Autodesk Fusion 360 part; units mm, degrees
(part 5 of 7)
sketch "Sketch2" plane through (0, 0, 2.4) normal (0, 0, 1) x (-1, 0, 0)
  circle A0 centre (0, 0) radius 8
  circle A1 centre (-15, 0) radius 5
  circle A2 centre (-4.6353, -14.2658) radius 5
  circle A3 centre (12.1353, -8.8168) radius 5
  circle A4 centre (12.1353, 8.8168) radius 5
  circle A5 centre (-4.6353, 14.2658) radius 5
  spline S0 degree 3 poles (-29.7434, 3.9157) (-29.7721, 3.6879) (-29.7146, 3.4878) (-29.6557, 3.3817) (-29.6311, 3.3373) (-29.6049, 3.3046) (-29.584, 3.2827) (-29.5723, 3.2703) (-29.5626, 3.2612) (-29.5043, 3.2074) (-29.4679, 3.1738) (-29.4161, 3.1342) (-29.3067, 3.0042) (-29.2288, 2.9117) (-29.097, 2.7401) (-29.0108, 2.4766) (-28.943, 2.2694) (-28.9321, 2.0574) (-28.9353, 1.9521) (-28.9382, 1.8554) (-28.9402, 1.7765) (-28.9853, 1.605) (-29.0418, 1.39) (-29.1868, 1.1346) (-29.3008, 0.9996) (-29.5122, 0.7494) (-29.5978, 0.7228) (-29.6536, 0.6831) (-29.7775, 0.595) (-29.758, 0.61) (-29.7843, 0.5851) (-29.8704, 0.5036) (-29.9984, 0.2947) (-30, -0.0001) knots 0.001251 0.001251 0.001251 0.001251 0.25 0.25 0.25 0.35404 0.35404 0.35404 0.412746 0.412746 0.412746 0.449449 0.449449 0.449449 0.475576 0.475576 0.475576 0.496118 0.496118 0.496118 0.514995 0.514995 0.514995 0.538647 0.538647 0.538647 0.582499 0.582499 0.582499 0.679826 0.679826 0.679826 0.99875 0.99875 0.99875 0.99875
  spline S1 degree 3 poles (-30, -0.0001) (-29.9988, -0.2297) (-29.9157, -0.4205) (-29.8434, -0.5181) (-29.8132, -0.5589) (-29.7829, -0.5878) (-29.7594, -0.6069) (-29.7462, -0.6177) (-29.7353, -0.6254) (-29.6705, -0.6711) (-29.63, -0.6997) (-29.5735, -0.7321) (-29.4481, -0.8468) (-29.3588, -0.9283) (-29.2058, -1.0812) (-29.0859, -1.3313) (-28.9916, -1.5279) (-28.9531, -1.7366) (-28.9425, -1.8414) (-28.9328, -1.9377) (-28.9245, -2.0161) (-28.9468, -2.1921) (-28.9748, -2.4126) (-29.0852, -2.6848) (-29.1806, -2.8335) (-29.3575, -3.1091) (-29.4389, -3.1467) (-29.4891, -3.1933) (-29.6004, -3.2968) (-29.583, -3.2795) (-29.6058, -3.3076) (-29.6806, -3.3996) (-29.7802, -3.6234) (-29.7433, -3.9159) knots 0.001251 0.001251 0.001251 0.001251 0.25 0.25 0.25 0.35404 0.35404 0.35404 0.412746 0.412746 0.412746 0.449449 0.449449 0.449449 0.475576 0.475576 0.475576 0.496118 0.496118 0.496118 0.514995 0.514995 0.514995 0.538647 0.538647 0.538647 0.582499 0.582499 0.582499 0.679826 0.679826 0.679826 0.99875 0.99875 0.99875 0.99875
  spline S2 degree 3 poles (-29.7433, -3.9159) (-29.7122, -4.1433) (-29.6048, -4.3217) (-29.5205, -4.409) (-29.4852, -4.4455) (-29.4514, -4.4703) (-29.4256, -4.4861) (-29.4111, -4.495) (-29.3993, -4.5013) (-29.3291, -4.5382) (-29.2852, -4.5612) (-29.2249, -4.586) (-29.0856, -4.6833) (-28.9864, -4.7525) (-28.8148, -4.8841) (-28.6632, -5.1164) (-28.5441, -5.299) (-28.4788, -5.5009) (-28.4546, -5.6034) (-28.4323, -5.6976) (-28.4139, -5.7743) (-28.413, -5.9517) (-28.412, -6.1739) (-28.4859, -6.4582) (-28.5611, -6.6181) (-28.7005, -6.9144) (-28.7764, -6.9623) (-28.82, -7.0151) (-28.9168, -7.1322) (-28.9019, -7.1128) (-28.9208, -7.1436) (-28.9829, -7.2446) (-29.0525, -7.4795) (-28.9777, -7.7647) knots 0.001251 0.001251 0.001251 0.001251 0.25 0.25 0.25 0.35404 0.35404 0.35404 0.412746 0.412746 0.412746 0.449449 0.449449 0.449449 0.475576 0.475576 0.475576 0.496118 0.496118 0.496118 0.514995 0.514995 0.514995 0.538647 0.538647 0.538647 0.582499 0.582499 0.582499 0.679826 0.679826 0.679826 0.99875 0.99875 0.99875 0.99875
  spline S3 degree 3 poles (-28.9777, -7.7647) (-28.9172, -7.9861) (-28.7875, -8.1489) (-28.6924, -8.2245) (-28.6527, -8.2561) (-28.616, -8.2762) (-28.5883, -8.2885) (-28.5727, -8.2955) (-28.5603, -8.3002) (-28.4858, -8.3276) (-28.4393, -8.3447) (-28.3763, -8.3614) (-28.2255, -8.4396) (-28.1181, -8.4953) (-27.9308, -8.6034) (-27.7502, -8.8139) (-27.6083, -8.9794) (-27.5171, -9.1711) (-27.4797, -9.2695) (-27.4454, -9.36) (-27.4171, -9.4336) (-27.3931, -9.6094) (-27.363, -9.8296) (-27.3993, -10.1211) (-27.4529, -10.2894) (-27.5525, -10.6015) (-27.6214, -10.6588) (-27.6578, -10.7168) (-27.7385, -10.8456) (-27.7262, -10.8244) (-27.741, -10.8574) (-27.7894, -10.9657) (-27.8277, -11.2076) (-27.7163, -11.4806) knots 0.001251 0.001251 0.001251 0.001251 0.25 0.25 0.25 0.35404 0.35404 0.35404 0.412746 0.412746 0.412746 0.449449 0.449449 0.449449 0.475576 0.475576 0.475576 0.496118 0.496118 0.496118 0.514995 0.514995 0.514995 0.538647 0.538647 0.538647 0.582499 0.582499 0.582499 0.679826 0.679826 0.679826 0.99875 0.99875 0.99875 0.99875
  spline S4 degree 3 poles (-27.7163, -11.4806) (-27.6274, -11.6922) (-27.4775, -11.8368) (-27.3735, -11.8992) (-27.3299, -11.9254) (-27.2909, -11.9405) (-27.2619, -11.9492) (-27.2455, -11.954) (-27.2325, -11.9571) (-27.1552, -11.9745) (-27.1068, -11.9853) (-27.0422, -11.9937) (-26.8824, -12.0516) (-26.7687, -12.0928) (-26.5688, -12.1755) (-26.3624, -12.3606) (-26.2, -12.5062) (-26.0846, -12.6843) (-26.0347, -12.7771) (-25.9889, -12.8623) (-25.9512, -12.9316) (-25.9045, -13.1027) (-25.8459, -13.3171) (-25.8438, -13.6108) (-25.875, -13.7847) (-25.933, -14.1071) (-25.9939, -14.173) (-26.0223, -14.2352) (-26.0856, -14.3734) (-26.0762, -14.3508) (-26.0865, -14.3854) (-26.1203, -14.4991) (-26.1267, -14.744) (-25.9807, -15.0001) knots 0.001251 0.001251 0.001251 0.001251 0.25 0.25 0.25 0.35404 0.35404 0.35404 0.412746 0.412746 0.412746 0.449449 0.449449 0.449449 0.475576 0.475576 0.475576 0.496118 0.496118 0.496118 0.514995 0.514995 0.514995 0.538647 0.538647 0.538647 0.582499 0.582499 0.582499 0.679826 0.679826 0.679826 0.99875 0.99875 0.99875 0.99875
  spline S5 degree 3 poles (-25.9807, -15.0001) (-25.8649, -15.1983) (-25.6975, -15.322) (-25.5861, -15.3704) (-25.5395, -15.3906) (-25.4989, -15.4006) (-25.469, -15.4053) (-25.4521, -15.408) (-25.4388, -15.4093) (-25.3599, -15.4165) (-25.3105, -15.421) (-25.2453, -15.4208) (-25.0794, -15.4573) (-24.9613, -15.4834) (-24.7523, -15.5393) (-24.5234, -15.6959) (-24.3435, -15.819) (-24.2058, -15.9805) (-24.1443, -16.066) (-24.0877, -16.1444) (-24.0413, -16.2082) (-23.9726, -16.3718) (-23.8866, -16.5767) (-23.8461, -16.8677) (-23.8544, -17.0441) (-23.8698, -17.3713) (-23.9215, -17.4446) (-23.9416, -17.51) (-23.9863, -17.6553) (-23.9799, -17.6316) (-23.9856, -17.6673) (-24.0044, -17.7844) (-23.9787, -18.028) (-23.8005, -18.2629) knots 0.001251 0.001251 0.001251 0.001251 0.25 0.25 0.25 0.35404 0.35404 0.35404 0.412746 0.412746 0.412746 0.449449 0.449449 0.449449 0.475576 0.475576 0.475576 0.496118 0.496118 0.496118 0.514995 0.514995 0.514995 0.538647 0.538647 0.538647 0.582499 0.582499 0.582499 0.679826 0.679826 0.679826 0.99875 0.99875 0.99875 0.99875
  spline S6 degree 3 poles (-23.8005, -18.2629) (-23.6598, -18.4443) (-23.4777, -18.5451) (-23.361, -18.5786) (-23.3122, -18.5925) (-23.2705, -18.5971) (-23.2403, -18.5979) (-23.2232, -18.5984) (-23.2099, -18.5979) (-23.1307, -18.5947) (-23.0811, -18.5927) (-23.0165, -18.5841) (-22.8472, -18.5986) (-22.7267, -18.609) (-22.5123, -18.6372) (-22.2649, -18.7625) (-22.0704, -18.8611) (-21.9129, -19.0033) (-21.8407, -19.08) (-21.7743, -19.1504) (-21.72, -19.2076) (-21.6306, -19.3608) (-21.5185, -19.5527) (-21.4404, -19.8359) (-21.4256, -20.012) (-21.3981, -20.3383) (-21.4399, -20.4177) (-21.4513, -20.4852) (-21.4766, -20.6351) (-21.4734, -20.6108) (-21.4744, -20.647) (-21.4777, -20.7655) (-21.4205, -21.0037) (-21.2131, -21.2133) knots 0.001251 0.001251 0.001251 0.001251 0.25 0.25 0.25 0.35404 0.35404 0.35404 0.412746 0.412746 0.412746 0.449449 0.449449 0.449449 0.475576 0.475576 0.475576 0.496118 0.496118 0.496118 0.514995 0.514995 0.514995 0.538647 0.538647 0.538647 0.582499 0.582499 0.582499 0.679826 0.679826 0.679826 0.99875 0.99875 0.99875 0.99875
  spline S7 degree 3 poles (-21.2131, -21.2133) (-21.05, -21.3747) (-20.8562, -21.4509) (-20.7361, -21.4688) (-20.6859, -21.4763) (-20.6441, -21.4754) (-20.6139, -21.4722) (-20.5969, -21.4705) (-20.5838, -21.4683) (-20.5057, -21.4548) (-20.4568, -21.4463) (-20.3939, -21.4293) (-20.2242, -21.4217) (-20.1033, -21.4162) (-19.887, -21.4162) (-19.6254, -21.5082) (-19.4198, -21.5805) (-19.245, -21.701) (-19.1634, -21.7675) (-19.0884, -21.8287) (-19.0271, -21.8783) (-18.9184, -22.0185) (-18.7823, -22.1942) (-18.6679, -22.4648) (-18.6302, -22.6374) (-18.5604, -22.9574) (-18.5914, -23.0415) (-18.5939, -23.1099) (-18.5994, -23.2618) (-18.5994, -23.2373) (-18.5957, -23.2733) (-18.5835, -23.3912) (-18.4957, -23.6199) (-18.2627, -23.8007) knots 0.001251 0.001251 0.001251 0.001251 0.25 0.25 0.25 0.35404 0.35404 0.35404 0.412746 0.412746 0.412746 0.449449 0.449449 0.449449 0.475576 0.475576 0.475576 0.496118 0.496118 0.496118 0.514995 0.514995 0.514995 0.538647 0.538647 0.538647 0.582499 0.582499 0.582499 0.679826 0.679826 0.679826 0.99875 0.99875 0.99875 0.99875
  spline S8 degree 3 poles (-18.2627, -23.8007) (-18.0799, -23.9394) (-17.8779, -23.9897) (-17.7565, -23.9918) (-17.7057, -23.9926) (-17.6643, -23.9862) (-17.6349, -23.9792) (-17.6183, -23.9752) (-17.6055, -23.9714) (-17.5298, -23.9478) (-17.4825, -23.933) (-17.4224, -23.908) (-17.2551, -23.8782) (-17.136, -23.857) (-16.9215, -23.8287) (-16.6502, -23.8858) (-16.4368, -23.9307) (-16.2478, -24.0273) (-16.1582, -24.0826) (-16.0759, -24.1335) (-16.0086, -24.1747) (-15.8826, -24.2995) (-15.7247, -24.4559) (-15.576, -24.7092) (-15.5161, -24.8754) (-15.4051, -25.1836) (-15.4249, -25.2711) (-15.4184, -25.3392) (-15.404, -25.4905) (-15.4072, -25.4662) (-15.3988, -25.5014) (-15.3713, -25.6167) (-15.2544, -25.832) (-14.9999, -25.9808) knots 0.001251 0.001251 0.001251 0.001251 0.25 0.25 0.25 0.35404 0.35404 0.35404 0.412746 0.412746 0.412746 0.449449 0.449449 0.449449 0.475576 0.475576 0.475576 0.496118 0.496118 0.496118 0.514995 0.514995 0.514995 0.538647 0.538647 0.538647 0.582499 0.582499 0.582499 0.679826 0.679826 0.679826 0.99875 0.99875 0.99875 0.99875
  spline S9 degree 3 poles (-14.9999, -25.9808) (-14.8005, -26.0945) (-14.5936, -26.118) (-14.473, -26.1042) (-14.4226, -26.0984) (-14.3824, -26.0867) (-14.3541, -26.0759) (-14.3382, -26.0698) (-14.326, -26.0643) (-14.2541, -26.031) (-14.2091, -26.0102) (-14.1527, -25.9775) (-13.9907, -25.9262) (-13.8754, -25.8896) (-13.6665, -25.8336) (-13.39, -25.8547) (-13.1726, -25.8714) (-12.9726, -25.9425) (-12.8766, -25.9857) (-12.7883, -26.0253) (-12.7162, -26.0574) (-12.575, -26.1647) (-12.398, -26.2992) (-12.2175, -26.5309) (-12.1364, -26.6879) (-11.9862, -26.9789) (-11.9944, -27.0682) (-11.9791, -27.135) (-11.9451, -27.2831) (-11.9514, -27.2594) (-11.9385, -27.2932) (-11.8962, -27.4039) (-11.7522, -27.6021) (-11.4804, -27.7164) knots 0.001251 0.001251 0.001251 0.001251 0.25 0.25 0.25 0.35404 0.35404 0.35404 0.412746 0.412746 0.412746 0.449449 0.449449 0.449449 0.475576 0.475576 0.475576 0.496118 0.496118 0.496118 0.514995 0.514995 0.514995 0.538647 0.538647 0.538647 0.582499 0.582499 0.582499 0.679826 0.679826 0.679826 0.99875 0.99875 0.99875 0.99875
  spline S10 degree 3 poles (-11.4804, -27.7164) (-11.2679, -27.8031) (-11.0597, -27.7994) (-10.9419, -27.77) (-10.8927, -27.7577) (-10.8543, -27.7408) (-10.8277, -27.7264) (-10.8127, -27.7182) (-10.8014, -27.7112) (-10.7344, -27.6688) (-10.6925, -27.6423) (-10.6409, -27.6025) (-10.487, -27.5305) (-10.3774, -27.4792) (-10.1776, -27.3964) (-9.9007, -27.3813) (-9.683, -27.3694) (-9.4754, -27.4138) (-9.3746, -27.4441) (-9.2819, -27.4719) (-9.2063, -27.4943) (-9.0522, -27.5822) (-8.8592, -27.6924) (-8.65, -27.8986) (-8.5492, -28.0437) (-8.3622, -28.3126) (-8.3586, -28.4022) (-8.3347, -28.4664) (-8.2817, -28.6088) (-8.2911, -28.5861) (-8.2739, -28.618) (-8.2175, -28.7223) (-8.0488, -28.8999) (-7.7644, -28.9778) knots 0.001251 0.001251 0.001251 0.001251 0.25 0.25 0.25 0.35404 0.35404 0.35404 0.412746 0.412746 0.412746 0.449449 0.449449 0.449449 0.475576 0.475576 0.475576 0.496118 0.496118 0.496118 0.514995 0.514995 0.514995 0.538647 0.538647 0.538647 0.582499 0.582499 0.582499 0.679826 0.679826 0.679826 0.99875 0.99875 0.99875 0.99875
  spline S11 degree 3 poles (-7.7644, -28.9778) (-7.5424, -29.036) (-7.3365, -29.0052) (-7.2236, -28.9606) (-7.1764, -28.942) (-7.1406, -28.9203) (-7.1161, -28.9025) (-7.1022, -28.8924) (-7.0919, -28.884) (-7.031, -28.8332) (-6.993, -28.8015) (-6.947, -28.7553) (-6.8038, -28.6638) (-6.7019, -28.5987) (-6.5146, -28.4905) (-6.242, -28.4393) (-6.0278, -28.3991) (-5.8162, -28.4161) (-5.7122, -28.4329) (-5.6167, -28.4484) (-5.5388, -28.4607) (-5.3746, -28.5278) (-5.1689, -28.6119) (-4.9345, -28.789) (-4.8156, -28.9196) (-4.5951, -29.1619) (-4.5799, -29.2503) (-4.5478, -29.3108) (-4.4767, -29.445) (-4.4889, -29.4238) (-4.4677, -29.4531) (-4.3982, -29.5491) (-4.2078, -29.7033) (-3.9157, -29.7434) knots 0.001251 0.001251 0.001251 0.001251 0.25 0.25 0.25 0.35404 0.35404 0.35404 0.412746 0.412746 0.412746 0.449449 0.449449 0.449449 0.475576 0.475576 0.475576 0.496118 0.496118 0.496118 0.514995 0.514995 0.514995 0.538647 0.538647 0.538647 0.582499 0.582499 0.582499 0.679826 0.679826 0.679826 0.99875 0.99875 0.99875 0.99875
  spline S12 degree 3 poles (-3.9157, -29.7434) (-3.6879, -29.7721) (-3.4878, -29.7146) (-3.3817, -29.6557) (-3.3373, -29.6311) (-3.3046, -29.6049) (-3.2827, -29.584) (-3.2703, -29.5723) (-3.2612, -29.5626) (-3.2074, -29.5043) (-3.1738, -29.4679) (-3.1342, -29.4161) (-3.0042, -29.3067) (-2.9117, -29.2288) (-2.7401, -29.097) (-2.4766, -29.0108) (-2.2694, -28.943) (-2.0574, -28.9321) (-1.9521, -28.9353) (-1.8554, -28.9382) (-1.7765, -28.9402) (-1.605, -28.9853) (-1.39, -29.0418) (-1.1346, -29.1868) (-0.9996, -29.3008) (-0.7494, -29.5122) (-0.7228, -29.5978) (-0.6831, -29.6536) (-0.595, -29.7775) (-0.61, -29.758) (-0.5851, -29.7843) (-0.5036, -29.8704) (-0.2947, -29.9984) (0.0001, -30) knots 0.001251 0.001251 0.001251 0.001251 0.25 0.25 0.25 0.35404 0.35404 0.35404 0.412746 0.412746 0.412746 0.449449 0.449449 0.449449 0.475576 0.475576 0.475576 0.496118 0.496118 0.496118 0.514995 0.514995 0.514995 0.538647 0.538647 0.538647 0.582499 0.582499 0.582499 0.679826 0.679826 0.679826 0.99875 0.99875 0.99875 0.99875
  spline S13 degree 3 poles (0.0001, -30) (0.2297, -29.9988) (0.4205, -29.9157) (0.5181, -29.8434) (0.5589, -29.8132) (0.5878, -29.7829) (0.6069, -29.7594) (0.6177, -29.7462) (0.6254, -29.7353) (0.6711, -29.6705) (0.6997, -29.63) (0.7321, -29.5735) (0.8468, -29.4481) (0.9283, -29.3588) (1.0812, -29.2058) (1.3313, -29.0859) (1.5279, -28.9916) (1.7366, -28.9531) (1.8414, -28.9425) (1.9377, -28.9328) (2.0161, -28.9245) (2.1921, -28.9468) (2.4126, -28.9748) (2.6848, -29.0852) (2.8335, -29.1806) (3.1091, -29.3575) (3.1467, -29.4389) (3.1933, -29.4891) (3.2968, -29.6004) (3.2795, -29.583) (3.3076, -29.6058) (3.3996, -29.6806) (3.6234, -29.7802) (3.9159, -29.7433) knots 0.001251 0.001251 0.001251 0.001251 0.25 0.25 0.25 0.35404 0.35404 0.35404 0.412746 0.412746 0.412746 0.449449 0.449449 0.449449 0.475576 0.475576 0.475576 0.496118 0.496118 0.496118 0.514995 0.514995 0.514995 0.538647 0.538647 0.538647 0.582499 0.582499 0.582499 0.679826 0.679826 0.679826 0.99875 0.99875 0.99875 0.99875
  spline S14 degree 3 poles (3.9159, -29.7433) (4.1433, -29.7122) (4.3217, -29.6048) (4.409, -29.5205) (4.4455, -29.4852) (4.4703, -29.4514) (4.4861, -29.4256) (4.495, -29.4111) (4.5013, -29.3993) (4.5382, -29.3291) (4.5612, -29.2852) (4.586, -29.2249) (4.6833, -29.0856) (4.7525, -28.9864) (4.8841, -28.8148) (5.1164, -28.6632) (5.299, -28.5441) (5.5009, -28.4788) (5.6034, -28.4546) (5.6976, -28.4323) (5.7743, -28.4139) (5.9517, -28.413) (6.1739, -28.412) (6.4582, -28.4859) (6.6181, -28.5611) (6.9144, -28.7005) (6.9623, -28.7764) (7.0151, -28.82) (7.1322, -28.9168) (7.1128, -28.9019) (7.1436, -28.9208) (7.2446, -28.9829) (7.4795, -29.0525) (7.7647, -28.9777) knots 0.001251 0.001251 0.001251 0.001251 0.25 0.25 0.25 0.35404 0.35404 0.35404 0.412746 0.412746 0.412746 0.449449 0.449449 0.449449 0.475576 0.475576 0.475576 0.496118 0.496118 0.496118 0.514995 0.514995 0.514995 0.538647 0.538647 0.538647 0.582499 0.582499 0.582499 0.679826 0.679826 0.679826 0.99875 0.99875 0.99875 0.99875
  spline S15 degree 3 poles (7.7647, -28.9777) (7.9861, -28.9172) (8.1489, -28.7875) (8.2245, -28.6924) (8.2561, -28.6527) (8.2762, -28.616) (8.2885, -28.5883) (8.2955, -28.5727) (8.3002, -28.5603) (8.3276, -28.4858) (8.3447, -28.4393) (8.3614, -28.3763) (8.4396, -28.2255) (8.4953, -28.1181) (8.6034, -27.9308) (8.8139, -27.7502) (8.9794, -27.6083) (9.1711, -27.5171) (9.2695, -27.4797) (9.36, -27.4454) (9.4336, -27.4171) (9.6094, -27.3931) (9.8296, -27.363) (10.1211, -27.3993) (10.2894, -27.4529) (10.6015, -27.5525) (10.6588, -27.6214) (10.7168, -27.6578) (10.8456, -27.7385) (10.8244, -27.7262) (10.8574, -27.741) (10.9657, -27.7894) (11.2076, -27.8277) (11.4806, -27.7163) knots 0.001251 0.001251 0.001251 0.001251 0.25 0.25 0.25 0.35404 0.35404 0.35404 0.412746 0.412746 0.412746 0.449449 0.449449 0.449449 0.475576 0.475576 0.475576 0.496118 0.496118 0.496118 0.514995 0.514995 0.514995 0.538647 0.538647 0.538647 0.582499 0.582499 0.582499 0.679826 0.679826 0.679826 0.99875 0.99875 0.99875 0.99875
  spline S16 degree 3 poles (11.4806, -27.7163) (11.6922, -27.6274) (11.8368, -27.4775) (11.8992, -27.3735) (11.9254, -27.3299) (11.9405, -27.2909) (11.9492, -27.2619) (11.954, -27.2455) (11.9571, -27.2325) (11.9745, -27.1552) (11.9853, -27.1068) (11.9937, -27.0422) (12.0516, -26.8824) (12.0928, -26.7687) (12.1755, -26.5688) (12.3606, -26.3624) (12.5062, -26.2) (12.6843, -26.0846) (12.7771, -26.0347) (12.8623, -25.9889) (12.9316, -25.9512) (13.1027, -25.9045) (13.3171, -25.8459) (13.6108, -25.8438) (13.7847, -25.875) (14.1071, -25.933) (14.173, -25.9939) (14.2352, -26.0223) (14.3734, -26.0856) (14.3508, -26.0762) (14.3854, -26.0865) (14.4991, -26.1203) (14.744, -26.1267) (15.0001, -25.9807) knots 0.001251 0.001251 0.001251 0.001251 0.25 0.25 0.25 0.35404 0.35404 0.35404 0.412746 0.412746 0.412746 0.449449 0.449449 0.449449 0.475576 0.475576 0.475576 0.496118 0.496118 0.496118 0.514995 0.514995 0.514995 0.538647 0.538647 0.538647 0.582499 0.582499 0.582499 0.679826 0.679826 0.679826 0.99875 0.99875 0.99875 0.99875
  spline S17 degree 3 poles (15.0001, -25.9807) (15.1983, -25.8649) (15.322, -25.6975) (15.3704, -25.5861) (15.3906, -25.5395) (15.4006, -25.4989) (15.4053, -25.469) (15.408, -25.4521) (15.4093, -25.4388) (15.4165, -25.3599) (15.421, -25.3105) (15.4208, -25.2453) (15.4573, -25.0794) (15.4834, -24.9613) (15.5393, -24.7523) (15.6959, -24.5234) (15.819, -24.3435) (15.9805, -24.2058) (16.066, -24.1443) (16.1444, -24.0877) (16.2082, -24.0413) (16.3718, -23.9726) (16.5767, -23.8866) (16.8677, -23.8461) (17.0441, -23.8544) (17.3713, -23.8698) (17.4446, -23.9215) (17.51, -23.9416) (17.6553, -23.9863) (17.6316, -23.9799) (17.6673, -23.9856) (17.7844, -24.0044) (18.028, -23.9787) (18.2629, -23.8005) knots 0.001251 0.001251 0.001251 0.001251 0.25 0.25 0.25 0.35404 0.35404 0.35404 0.412746 0.412746 0.412746 0.449449 0.449449 0.449449 0.475576 0.475576 0.475576 0.496118 0.496118 0.496118 0.514995 0.514995 0.514995 0.538647 0.538647 0.538647 0.582499 0.582499 0.582499 0.679826 0.679826 0.679826 0.99875 0.99875 0.99875 0.99875
  spline S18 degree 3 poles (18.2629, -23.8005) (18.4443, -23.6598) (18.5451, -23.4777) (18.5786, -23.361) (18.5925, -23.3122) (18.5971, -23.2705) (18.5979, -23.2403) (18.5984, -23.2232) (18.5979, -23.2099) (18.5947, -23.1307) (18.5927, -23.0811) (18.5841, -23.0165) (18.5986, -22.8472) (18.609, -22.7267) (18.6372, -22.5123) (18.7625, -22.2649) (18.8611, -22.0704) (19.0033, -21.9129) (19.08, -21.8407) (19.1504, -21.7743) (19.2076, -21.72) (19.3608, -21.6306) (19.5527, -21.5185) (19.8359, -21.4404) (20.012, -21.4256) (20.3383, -21.3981) (20.4177, -21.4399) (20.4852, -21.4513) (20.6351, -21.4766) (20.6108, -21.4734) (20.647, -21.4744) (20.7655, -21.4777) (21.0037, -21.4205) (21.2133, -21.2131) knots 0.001251 0.001251 0.001251 0.001251 0.25 0.25 0.25 0.35404 0.35404 0.35404 0.412746 0.412746 0.412746 0.449449 0.449449 0.449449 0.475576 0.475576 0.475576 0.496118 0.496118 0.496118 0.514995 0.514995 0.514995 0.538647 0.538647 0.538647 0.582499 0.582499 0.582499 0.679826 0.679826 0.679826 0.99875 0.99875 0.99875 0.99875
  spline S19 degree 3 poles (21.2133, -21.2131) (21.3747, -21.05) (21.4509, -20.8562) (21.4688, -20.7361) (21.4763, -20.6859) (21.4754, -20.6441) (21.4722, -20.6139) (21.4705, -20.5969) (21.4683, -20.5838) (21.4548, -20.5057) (21.4463, -20.4568) (21.4293, -20.3939) (21.4217, -20.2242) (21.4162, -20.1033) (21.4162, -19.887) (21.5082, -19.6254) (21.5805, -19.4198) (21.701, -19.245) (21.7675, -19.1634) (21.8287, -19.0884) (21.8783, -19.0271) (22.0185, -18.9184) (22.1942, -18.7823) (22.4648, -18.6679) (22.6374, -18.6302) (22.9574, -18.5604) (23.0415, -18.5914) (23.1099, -18.5939) (23.2618, -18.5994) (23.2373, -18.5994) (23.2733, -18.5957) (23.3912, -18.5835) (23.6199, -18.4957) (23.8007, -18.2627) knots 0.001251 0.001251 0.001251 0.001251 0.25 0.25 0.25 0.35404 0.35404 0.35404 0.412746 0.412746 0.412746 0.449449 0.449449 0.449449 0.475576 0.475576 0.475576 0.496118 0.496118 0.496118 0.514995 0.514995 0.514995 0.538647 0.538647 0.538647 0.582499 0.582499 0.582499 0.679826 0.679826 0.679826 0.99875 0.99875 0.99875 0.99875
  spline S20 degree 3 poles (23.8007, -18.2627) (23.9394, -18.0799) (23.9897, -17.8779) (23.9918, -17.7565) (23.9926, -17.7057) (23.9862, -17.6643) (23.9792, -17.6349) (23.9752, -17.6183) (23.9714, -17.6055) (23.9478, -17.5298) (23.933, -17.4825) (23.908, -17.4224) (23.8782, -17.2551) (23.857, -17.136) (23.8287, -16.9215) (23.8858, -16.6502) (23.9307, -16.4368) (24.0273, -16.2478) (24.0826, -16.1582) (24.1335, -16.0759) (24.1747, -16.0086) (24.2995, -15.8826) (24.4559, -15.7247) (24.7092, -15.576) (24.8754, -15.5161) (25.1836, -15.4051) (25.2711, -15.4249) (25.3392, -15.4184) (25.4905, -15.404) (25.4662, -15.4072) (25.5014, -15.3988) (25.6167, -15.3713) (25.832, -15.2544) (25.9808, -14.9999) knots 0.001251 0.001251 0.001251 0.001251 0.25 0.25 0.25 0.35404 0.35404 0.35404 0.412746 0.412746 0.412746 0.449449 0.449449 0.449449 0.475576 0.475576 0.475576 0.496118 0.496118 0.496118 0.514995 0.514995 0.514995 0.538647 0.538647 0.538647 0.582499 0.582499 0.582499 0.679826 0.679826 0.679826 0.99875 0.99875 0.99875 0.99875
  spline S21 degree 3 poles (25.9808, -14.9999) (26.0945, -14.8005) (26.118, -14.5936) (26.1042, -14.473) (26.0984, -14.4226) (26.0867, -14.3824) (26.0759, -14.3541) (26.0698, -14.3382) (26.0643, -14.326) (26.031, -14.2541) (26.0102, -14.2091) (25.9775, -14.1527) (25.9262, -13.9907) (25.8896, -13.8754) (25.8336, -13.6665) (25.8547, -13.39) (25.8714, -13.1726) (25.9425, -12.9726) (25.9857, -12.8766) (26.0253, -12.7883) (26.0574, -12.7162) (26.1647, -12.575) (26.2992, -12.398) (26.5309, -12.2175) (26.6879, -12.1364) (26.9789, -11.9862) (27.0682, -11.9944) (27.135, -11.9791) (27.2831, -11.9451) (27.2594, -11.9514) (27.2932, -11.9385) (27.4039, -11.8962) (27.6021, -11.7522) (27.7164, -11.4804) knots 0.001251 0.001251 0.001251 0.001251 0.25 0.25 0.25 0.35404 0.35404 0.35404 0.412746 0.412746 0.412746 0.449449 0.449449 0.449449 0.475576 0.475576 0.475576 0.496118 0.496118 0.496118 0.514995 0.514995 0.514995 0.538647 0.538647 0.538647 0.582499 0.582499 0.582499 0.679826 0.679826 0.679826 0.99875 0.99875 0.99875 0.99875
  spline S22 degree 3 poles (27.7164, -11.4804) (27.8031, -11.2679) (27.7994, -11.0597) (27.77, -10.9419) (27.7577, -10.8927) (27.7408, -10.8543) (27.7264, -10.8277) (27.7182, -10.8127) (27.7112, -10.8014) (27.6688, -10.7344) (27.6423, -10.6925) (27.6025, -10.6409) (27.5305, -10.487) (27.4792, -10.3774) (27.3964, -10.1776) (27.3813, -9.9007) (27.3694, -9.683) (27.4138, -9.4754) (27.4441, -9.3746) (27.4719, -9.2819) (27.4943, -9.2063) (27.5822, -9.0522) (27.6924, -8.8592) (27.8986, -8.65) (28.0437, -8.5492) (28.3126, -8.3622) (28.4022, -8.3586) (28.4664, -8.3347) (28.6088, -8.2817) (28.5861, -8.2911) (28.618, -8.2739) (28.7223, -8.2175) (28.8999, -8.0488) (28.9778, -7.7644) knots 0.001251 0.001251 0.001251 0.001251 0.25 0.25 0.25 0.35404 0.35404 0.35404 0.412746 0.412746 0.412746 0.449449 0.449449 0.449449 0.475576 0.475576 0.475576 0.496118 0.496118 0.496118 0.514995 0.514995 0.514995 0.538647 0.538647 0.538647 0.582499 0.582499 0.582499 0.679826 0.679826 0.679826 0.99875 0.99875 0.99875 0.99875
  spline S23 degree 3 poles (28.9778, -7.7644) (29.036, -7.5424) (29.0052, -7.3365) (28.9606, -7.2236) (28.942, -7.1764) (28.9203, -7.1406) (28.9025, -7.1161) (28.8924, -7.1022) (28.884, -7.0919) (28.8332, -7.031) (28.8015, -6.993) (28.7553, -6.947) (28.6638, -6.8038) (28.5987, -6.7019) (28.4905, -6.5146) (28.4393, -6.242) (28.3991, -6.0278) (28.4161, -5.8162) (28.4329, -5.7122) (28.4484, -5.6167) (28.4607, -5.5388) (28.5278, -5.3746) (28.6119, -5.1689) (28.789, -4.9345) (28.9196, -4.8156) (29.1619, -4.5951) (29.2503, -4.5799) (29.3108, -4.5478) (29.445, -4.4767) (29.4238, -4.4889) (29.4531, -4.4677) (29.5491, -4.3982) (29.7033, -4.2078) (29.7434, -3.9157) knots 0.001251 0.001251 0.001251 0.001251 0.25 0.25 0.25 0.35404 0.35404 0.35404 0.412746 0.412746 0.412746 0.449449 0.449449 0.449449 0.475576 0.475576 0.475576 0.496118 0.496118 0.496118 0.514995 0.514995 0.514995 0.538647 0.538647 0.538647 0.582499 0.582499 0.582499 0.679826 0.679826 0.679826 0.99875 0.99875 0.99875 0.99875
  spline S24 degree 3 poles (29.7434, -3.9157) (29.7721, -3.6879) (29.7146, -3.4878) (29.6557, -3.3817) (29.6311, -3.3373) (29.6049, -3.3046) (29.584, -3.2827) (29.5723, -3.2703) (29.5626, -3.2612) (29.5043, -3.2074) (29.4679, -3.1738) (29.4161, -3.1342) (29.3067, -3.0042) (29.2288, -2.9117) (29.097, -2.7401) (29.0108, -2.4766) (28.943, -2.2694) (28.9321, -2.0574) (28.9353, -1.9521) (28.9382, -1.8554) (28.9402, -1.7765) (28.9853, -1.605) (29.0418, -1.39) (29.1868, -1.1346) (29.3008, -0.9996) (29.5122, -0.7494) (29.5978, -0.7228) (29.6536, -0.6831) (29.7775, -0.595) (29.758, -0.61) (29.7843, -0.5851) (29.8704, -0.5036) (29.9984, -0.2947) (30, 0.0001) knots 0.001251 0.001251 0.001251 0.001251 0.25 0.25 0.25 0.35404 0.35404 0.35404 0.412746 0.412746 0.412746 0.449449 0.449449 0.449449 0.475576 0.475576 0.475576 0.496118 0.496118 0.496118 0.514995 0.514995 0.514995 0.538647 0.538647 0.538647 0.582499 0.582499 0.582499 0.679826 0.679826 0.679826 0.99875 0.99875 0.99875 0.99875
  spline S25 degree 3 poles (30, 0.0001) (29.9988, 0.2297) (29.9157, 0.4205) (29.8434, 0.5181) (29.8132, 0.5589) (29.7829, 0.5878) (29.7594, 0.6069) (29.7462, 0.6177) (29.7353, 0.6254) (29.6705, 0.6711) (29.63, 0.6997) (29.5735, 0.7321) (29.4481, 0.8468) (29.3588, 0.9283) (29.2058, 1.0812) (29.0859, 1.3313) (28.9916, 1.5279) (28.9531, 1.7366) (28.9425, 1.8414) (28.9328, 1.9377) (28.9245, 2.0161) (28.9468, 2.1921) (28.9748, 2.4126) (29.0852, 2.6848) (29.1806, 2.8335) (29.3575, 3.1091) (29.4389, 3.1467) (29.4891, 3.1933) (29.6004, 3.2968) (29.583, 3.2795) (29.6058, 3.3076) (29.6806, 3.3996) (29.7802, 3.6234) (29.7433, 3.9159) knots 0.001251 0.001251 0.001251 0.001251 0.25 0.25 0.25 0.35404 0.35404 0.35404 0.412746 0.412746 0.412746 0.449449 0.449449 0.449449 0.475576 0.475576 0.475576 0.496118 0.496118 0.496118 0.514995 0.514995 0.514995 0.538647 0.538647 0.538647 0.582499 0.582499 0.582499 0.679826 0.679826 0.679826 0.99875 0.99875 0.99875 0.99875
  spline S26 degree 3 poles (29.7433, 3.9159) (29.7122, 4.1433) (29.6048, 4.3217) (29.5205, 4.409) (29.4852, 4.4455) (29.4514, 4.4703) (29.4256, 4.4861) (29.4111, 4.495) (29.3993, 4.5013) (29.3291, 4.5382) (29.2852, 4.5612) (29.2249, 4.586) (29.0856, 4.6833) (28.9864, 4.7525) (28.8148, 4.8841) (28.6632, 5.1164) (28.5441, 5.299) (28.4788, 5.5009) (28.4546, 5.6034) (28.4323, 5.6976) (28.4139, 5.7743) (28.413, 5.9517) (28.412, 6.1739) (28.4859, 6.4582) (28.5611, 6.6181) (28.7005, 6.9144) (28.7764, 6.9623) (28.82, 7.0151) (28.9168, 7.1322) (28.9019, 7.1128) (28.9208, 7.1436) (28.9829, 7.2446) (29.0525, 7.4795) (28.9777, 7.7647) knots 0.001251 0.001251 0.001251 0.001251 0.25 0.25 0.25 0.35404 0.35404 0.35404 0.412746 0.412746 0.412746 0.449449 0.449449 0.449449 0.475576 0.475576 0.475576 0.496118 0.496118 0.496118 0.514995 0.514995 0.514995 0.538647 0.538647 0.538647 0.582499 0.582499 0.582499 0.679826 0.679826 0.679826 0.99875 0.99875 0.99875 0.99875
  spline S27 degree 3 poles (28.9777, 7.7647) (28.9172, 7.9861) (28.7875, 8.1489) (28.6924, 8.2245) (28.6527, 8.2561) (28.616, 8.2762) (28.5883, 8.2885) (28.5727, 8.2955) (28.5603, 8.3002) (28.4858, 8.3276) (28.4393, 8.3447) (28.3763, 8.3614) (28.2255, 8.4396) (28.1181, 8.4953) (27.9308, 8.6034) (27.7502, 8.8139) (27.6083, 8.9794) (27.5171, 9.1711) (27.4797, 9.2695) (27.4454, 9.36) (27.4171, 9.4336) (27.3931, 9.6094) (27.363, 9.8296) (27.3993, 10.1211) (27.4529, 10.2894) (27.5525, 10.6015) (27.6214, 10.6588) (27.6578, 10.7168) (27.7385, 10.8456) (27.7262, 10.8244) (27.741, 10.8574) (27.7894, 10.9657) (27.8277, 11.2076) (27.7163, 11.4806) knots 0.001251 0.001251 0.001251 0.001251 0.25 0.25 0.25 0.35404 0.35404 0.35404 0.412746 0.412746 0.412746 0.449449 0.449449 0.449449 0.475576 0.475576 0.475576 0.496118 0.496118 0.496118 0.514995 0.514995 0.514995 0.538647 0.538647 0.538647 0.582499 0.582499 0.582499 0.679826 0.679826 0.679826 0.99875 0.99875 0.99875 0.99875
  spline S28 degree 3 poles (27.7163, 11.4806) (27.6274, 11.6922) (27.4775, 11.8368) (27.3735, 11.8992) (27.3299, 11.9254) (27.2909, 11.9405) (27.2619, 11.9492) (27.2455, 11.954) (27.2325, 11.9571) (27.1552, 11.9745) (27.1068, 11.9853) (27.0422, 11.9937) (26.8824, 12.0516) (26.7687, 12.0928) (26.5688, 12.1755) (26.3624, 12.3606) (26.2, 12.5062) (26.0846, 12.6843) (26.0347, 12.7771) (25.9889, 12.8623) (25.9512, 12.9316) (25.9045, 13.1027) (25.8459, 13.3171) (25.8438, 13.6108) (25.875, 13.7847) (25.933, 14.1071) (25.9939, 14.173) (26.0223, 14.2352) (26.0856, 14.3734) (26.0762, 14.3508) (26.0865, 14.3854) (26.1203, 14.4991) (26.1267, 14.744) (25.9807, 15.0001) knots 0.001251 0.001251 0.001251 0.001251 0.25 0.25 0.25 0.35404 0.35404 0.35404 0.412746 0.412746 0.412746 0.449449 0.449449 0.449449 0.475576 0.475576 0.475576 0.496118 0.496118 0.496118 0.514995 0.514995 0.514995 0.538647 0.538647 0.538647 0.582499 0.582499 0.582499 0.679826 0.679826 0.679826 0.99875 0.99875 0.99875 0.99875
  spline S29 degree 3 poles (25.9807, 15.0001) (25.8649, 15.1983) (25.6975, 15.322) (25.5861, 15.3704) (25.5395, 15.3906) (25.4989, 15.4006) (25.469, 15.4053) (25.4521, 15.408) (25.4388, 15.4093) (25.3599, 15.4165) (25.3105, 15.421) (25.2453, 15.4208) (25.0794, 15.4573) (24.9613, 15.4834) (24.7523, 15.5393) (24.5234, 15.6959) (24.3435, 15.819) (24.2058, 15.9805) (24.1443, 16.066) (24.0877, 16.1444) (24.0413, 16.2082) (23.9726, 16.3718) (23.8866, 16.5767) (23.8461, 16.8677) (23.8544, 17.0441) (23.8698, 17.3713) (23.9215, 17.4446) (23.9416, 17.51) (23.9863, 17.6553) (23.9799, 17.6316) (23.9856, 17.6673) (24.0044, 17.7844) (23.9787, 18.028) (23.8005, 18.2629) knots 0.001251 0.001251 0.001251 0.001251 0.25 0.25 0.25 0.35404 0.35404 0.35404 0.412746 0.412746 0.412746 0.449449 0.449449 0.449449 0.475576 0.475576 0.475576 0.496118 0.496118 0.496118 0.514995 0.514995 0.514995 0.538647 0.538647 0.538647 0.582499 0.582499 0.582499 0.679826 0.679826 0.679826 0.99875 0.99875 0.99875 0.99875
  spline S30 degree 3 poles (23.8005, 18.2629) (23.6598, 18.4443) (23.4777, 18.5451) (23.361, 18.5786) (23.3122, 18.5925) (23.2705, 18.5971) (23.2403, 18.5979) (23.2232, 18.5984) (23.2099, 18.5979) (23.1307, 18.5947) (23.0811, 18.5927) (23.0165, 18.5841) (22.8472, 18.5986) (22.7267, 18.609) (22.5123, 18.6372) (22.2649, 18.7625) (22.0704, 18.8611) (21.9129, 19.0033) (21.8407, 19.08) (21.7743, 19.1504) (21.72, 19.2076) (21.6306, 19.3608) (21.5185, 19.5527) (21.4404, 19.8359) (21.4256, 20.012) (21.3981, 20.3383) (21.4399, 20.4177) (21.4513, 20.4852) (21.4766, 20.6351) (21.4734, 20.6108) (21.4744, 20.647) (21.4777, 20.7655) (21.4205, 21.0037) (21.2131, 21.2133) knots 0.001251 0.001251 0.001251 0.001251 0.25 0.25 0.25 0.35404 0.35404 0.35404 0.412746 0.412746 0.412746 0.449449 0.449449 0.449449 0.475576 0.475576 0.475576 0.496118 0.496118 0.496118 0.514995 0.514995 0.514995 0.538647 0.538647 0.538647 0.582499 0.582499 0.582499 0.679826 0.679826 0.679826 0.99875 0.99875 0.99875 0.99875
  spline S31 degree 3 poles (21.2131, 21.2133) (21.05, 21.3747) (20.8562, 21.4509) (20.7361, 21.4688) (20.6859, 21.4763) (20.6441, 21.4754) (20.6139, 21.4722) (20.5969, 21.4705) (20.5838, 21.4683) (20.5057, 21.4548) (20.4568, 21.4463) (20.3939, 21.4293) (20.2242, 21.4217) (20.1033, 21.4162) (19.887, 21.4162) (19.6254, 21.5082) (19.4198, 21.5805) (19.245, 21.701) (19.1634, 21.7675) (19.0884, 21.8287) (19.0271, 21.8783) (18.9184, 22.0185) (18.7823, 22.1942) (18.6679, 22.4648) (18.6302, 22.6374) (18.5604, 22.9574) (18.5914, 23.0415) (18.5939, 23.1099) (18.5994, 23.2618) (18.5994, 23.2373) (18.5957, 23.2733) (18.5835, 23.3912) (18.4957, 23.6199) (18.2627, 23.8007) knots 0.001251 0.001251 0.001251 0.001251 0.25 0.25 0.25 0.35404 0.35404 0.35404 0.412746 0.412746 0.412746 0.449449 0.449449 0.449449 0.475576 0.475576 0.475576 0.496118 0.496118 0.496118 0.514995 0.514995 0.514995 0.538647 0.538647 0.538647 0.582499 0.582499 0.582499 0.679826 0.679826 0.679826 0.99875 0.99875 0.99875 0.99875
  spline S32 degree 3 poles (18.2627, 23.8007) (18.0799, 23.9394) (17.8779, 23.9897) (17.7565, 23.9918) (17.7057, 23.9926) (17.6643, 23.9862) (17.6349, 23.9792) (17.6183, 23.9752) (17.6055, 23.9714) (17.5298, 23.9478) (17.4825, 23.933) (17.4224, 23.908) (17.2551, 23.8782) (17.136, 23.857) (16.9215, 23.8287) (16.6502, 23.8858) (16.4368, 23.9307) (16.2478, 24.0273) (16.1582, 24.0826) (16.0759, 24.1335) (16.0086, 24.1747) (15.8826, 24.2995) (15.7247, 24.4559) (15.576, 24.7092) (15.5161, 24.8754) (15.4051, 25.1836) (15.4249, 25.2711) (15.4184, 25.3392) (15.404, 25.4905) (15.4072, 25.4662) (15.3988, 25.5014) (15.3713, 25.6167) (15.2544, 25.832) (14.9999, 25.9808) knots 0.001251 0.001251 0.001251 0.001251 0.25 0.25 0.25 0.35404 0.35404 0.35404 0.412746 0.412746 0.412746 0.449449 0.449449 0.449449 0.475576 0.475576 0.475576 0.496118 0.496118 0.496118 0.514995 0.514995 0.514995 0.538647 0.538647 0.538647 0.582499 0.582499 0.582499 0.679826 0.679826 0.679826 0.99875 0.99875 0.99875 0.99875
  spline S33 degree 3 poles (14.9999, 25.9808) (14.8005, 26.0945) (14.5936, 26.118) (14.473, 26.1042) (14.4226, 26.0984) (14.3824, 26.0867) (14.3541, 26.0759) (14.3382, 26.0698) (14.326, 26.0643) (14.2541, 26.031) (14.2091, 26.0102) (14.1527, 25.9775) (13.9907, 25.9262) (13.8754, 25.8896) (13.6665, 25.8336) (13.39, 25.8547) (13.1726, 25.8714) (12.9726, 25.9425) (12.8766, 25.9857) (12.7883, 26.0253) (12.7162, 26.0574) (12.575, 26.1647) (12.398, 26.2992) (12.2175, 26.5309) (12.1364, 26.6879) (11.9862, 26.9789) (11.9944, 27.0682) (11.9791, 27.135) (11.9451, 27.2831) (11.9514, 27.2594) (11.9385, 27.2932) (11.8962, 27.4039) (11.7522, 27.6021) (11.4804, 27.7164) knots 0.001251 0.001251 0.001251 0.001251 0.25 0.25 0.25 0.35404 0.35404 0.35404 0.412746 0.412746 0.412746 0.449449 0.449449 0.449449 0.475576 0.475576 0.475576 0.496118 0.496118 0.496118 0.514995 0.514995 0.514995 0.538647 0.538647 0.538647 0.582499 0.582499 0.582499 0.679826 0.679826 0.679826 0.99875 0.99875 0.99875 0.99875
  spline S34 degree 3 poles (11.4804, 27.7164) (11.2679, 27.8031) (11.0597, 27.7994) (10.9419, 27.77) (10.8927, 27.7577) (10.8543, 27.7408) (10.8277, 27.7264) (10.8127, 27.7182) (10.8014, 27.7112) (10.7344, 27.6688) (10.6925, 27.6423) (10.6409, 27.6025) (10.487, 27.5305) (10.3774, 27.4792) (10.1776, 27.3964) (9.9007, 27.3813) (9.683, 27.3694) (9.4754, 27.4138) (9.3746, 27.4441) (9.2819, 27.4719) (9.2063, 27.4943) (9.0522, 27.5822) (8.8592, 27.6924) (8.65, 27.8986) (8.5492, 28.0437) (8.3622, 28.3126) (8.3586, 28.4022) (8.3347, 28.4664) (8.2817, 28.6088) (8.2911, 28.5861) (8.2739, 28.618) (8.2175, 28.7223) (8.0488, 28.8999) (7.7644, 28.9778) knots 0.001251 0.001251 0.001251 0.001251 0.25 0.25 0.25 0.35404 0.35404 0.35404 0.412746 0.412746 0.412746 0.449449 0.449449 0.449449 0.475576 0.475576 0.475576 0.496118 0.496118 0.496118 0.514995 0.514995 0.514995 0.538647 0.538647 0.538647 0.582499 0.582499 0.582499 0.679826 0.679826 0.679826 0.99875 0.99875 0.99875 0.99875
  spline S35 degree 3 poles (7.7644, 28.9778) (7.5424, 29.036) (7.3365, 29.0052) (7.2236, 28.9606) (7.1764, 28.942) (7.1406, 28.9203) (7.1161, 28.9025) (7.1022, 28.8924) (7.0919, 28.884) (7.031, 28.8332) (6.993, 28.8015) (6.947, 28.7553) (6.8038, 28.6638) (6.7019, 28.5987) (6.5146, 28.4905) (6.242, 28.4393) (6.0278, 28.3991) (5.8162, 28.4161) (5.7122, 28.4329) (5.6167, 28.4484) (5.5388, 28.4607) (5.3746, 28.5278) (5.1689, 28.6119) (4.9345, 28.789) (4.8156, 28.9196) (4.5951, 29.1619) (4.5799, 29.2503) (4.5478, 29.3108) (4.4767, 29.445) (4.4889, 29.4238) (4.4677, 29.4531) (4.3982, 29.5491) (4.2078, 29.7033) (3.9157, 29.7434) knots 0.001251 0.001251 0.001251 0.001251 0.25 0.25 0.25 0.35404 0.35404 0.35404 0.412746 0.412746 0.412746 0.449449 0.449449 0.449449 0.475576 0.475576 0.475576 0.496118 0.496118 0.496118 0.514995 0.514995 0.514995 0.538647 0.538647 0.538647 0.582499 0.582499 0.582499 0.679826 0.679826 0.679826 0.99875 0.99875 0.99875 0.99875
  spline S36 degree 3 poles (3.9157, 29.7434) (3.6879, 29.7721) (3.4878, 29.7146) (3.3817, 29.6557) (3.3373, 29.6311) (3.3046, 29.6049) (3.2827, 29.584) (3.2703, 29.5723) (3.2612, 29.5626) (3.2074, 29.5043) (3.1738, 29.4679) (3.1342, 29.4161) (3.0042, 29.3067) (2.9117, 29.2288) (2.7401, 29.097) (2.4766, 29.0108) (2.2694, 28.943) (2.0574, 28.9321) (1.9521, 28.9353) (1.8554, 28.9382) (1.7765, 28.9402) (1.605, 28.9853) (1.39, 29.0418) (1.1346, 29.1868) (0.9996, 29.3008) (0.7494, 29.5122) (0.7228, 29.5978) (0.6831, 29.6536) (0.595, 29.7775) (0.61, 29.758) (0.5851, 29.7843) (0.5036, 29.8704) (0.2947, 29.9984) (-0.0001, 30) knots 0.001251 0.001251 0.001251 0.001251 0.25 0.25 0.25 0.35404 0.35404 0.35404 0.412746 0.412746 0.412746 0.449449 0.449449 0.449449 0.475576 0.475576 0.475576 0.496118 0.496118 0.496118 0.514995 0.514995 0.514995 0.538647 0.538647 0.538647 0.582499 0.582499 0.582499 0.679826 0.679826 0.679826 0.99875 0.99875 0.99875 0.99875
  spline S37 degree 3 poles (-0.0001, 30) (-0.2297, 29.9988) (-0.4205, 29.9157) (-0.5181, 29.8434) (-0.5589, 29.8132) (-0.5878, 29.7829) (-0.6069, 29.7594) (-0.6177, 29.7462) (-0.6254, 29.7353) (-0.6711, 29.6705) (-0.6997, 29.63) (-0.7321, 29.5735) (-0.8468, 29.4481) (-0.9283, 29.3588) (-1.0812, 29.2058) (-1.3313, 29.0859) (-1.5279, 28.9916) (-1.7366, 28.9531) (-1.8414, 28.9425) (-1.9377, 28.9328) (-2.0161, 28.9245) (-2.1921, 28.9468) (-2.4126, 28.9748) (-2.6848, 29.0852) (-2.8335, 29.1806) (-3.1091, 29.3575) (-3.1467, 29.4389) (-3.1933, 29.4891) (-3.2968, 29.6004) (-3.2795, 29.583) (-3.3076, 29.6058) (-3.3996, 29.6806) (-3.6234, 29.7802) (-3.9159, 29.7433) knots 0.001251 0.001251 0.001251 0.001251 0.25 0.25 0.25 0.35404 0.35404 0.35404 0.412746 0.412746 0.412746 0.449449 0.449449 0.449449 0.475576 0.475576 0.475576 0.496118 0.496118 0.496118 0.514995 0.514995 0.514995 0.538647 0.538647 0.538647 0.582499 0.582499 0.582499 0.679826 0.679826 0.679826 0.99875 0.99875 0.99875 0.99875
  spline S38 degree 3 poles (-3.9159, 29.7433) (-4.1433, 29.7122) (-4.3217, 29.6048) (-4.409, 29.5205) (-4.4455, 29.4852) (-4.4703, 29.4514) (-4.4861, 29.4256) (-4.495, 29.4111) (-4.5013, 29.3993) (-4.5382, 29.3291) (-4.5612, 29.2852) (-4.586, 29.2249) (-4.6833, 29.0856) (-4.7525, 28.9864) (-4.8841, 28.8148) (-5.1164, 28.6632) (-5.299, 28.5441) (-5.5009, 28.4788) (-5.6034, 28.4546) (-5.6976, 28.4323) (-5.7743, 28.4139) (-5.9517, 28.413) (-6.1739, 28.412) (-6.4582, 28.4859) (-6.6181, 28.5611) (-6.9144, 28.7005) (-6.9623, 28.7764) (-7.0151, 28.82) (-7.1322, 28.9168) (-7.1128, 28.9019) (-7.1436, 28.9208) (-7.2446, 28.9829) (-7.4795, 29.0525) (-7.7647, 28.9777) knots 0.001251 0.001251 0.001251 0.001251 0.25 0.25 0.25 0.35404 0.35404 0.35404 0.412746 0.412746 0.412746 0.449449 0.449449 0.449449 0.475576 0.475576 0.475576 0.496118 0.496118 0.496118 0.514995 0.514995 0.514995 0.538647 0.538647 0.538647 0.582499 0.582499 0.582499 0.679826 0.679826 0.679826 0.99875 0.99875 0.99875 0.99875
  spline S39 degree 3 poles (-7.7647, 28.9777) (-7.9861, 28.9172) (-8.1489, 28.7875) (-8.2245, 28.6924) (-8.2561, 28.6527) (-8.2762, 28.616) (-8.2885, 28.5883) (-8.2955, 28.5727) (-8.3002, 28.5603) (-8.3276, 28.4858) (-8.3447, 28.4393) (-8.3614, 28.3763) (-8.4396, 28.2255) (-8.4953, 28.1181) (-8.6034, 27.9308) (-8.8139, 27.7502) (-8.9794, 27.6083) (-9.1711, 27.5171) (-9.2695, 27.4797) (-9.36, 27.4454) (-9.4336, 27.4171) (-9.6094, 27.3931) (-9.8296, 27.363) (-10.1211, 27.3993) (-10.2894, 27.4529) (-10.6015, 27.5525) (-10.6588, 27.6214) (-10.7168, 27.6578) (-10.8456, 27.7385) (-10.8244, 27.7262) (-10.8574, 27.741) (-10.9657, 27.7894) (-11.2076, 27.8277) (-11.4806, 27.7163) knots 0.001251 0.001251 0.001251 0.001251 0.25 0.25 0.25 0.35404 0.35404 0.35404 0.412746 0.412746 0.412746 0.449449 0.449449 0.449449 0.475576 0.475576 0.475576 0.496118 0.496118 0.496118 0.514995 0.514995 0.514995 0.538647 0.538647 0.538647 0.582499 0.582499 0.582499 0.679826 0.679826 0.679826 0.99875 0.99875 0.99875 0.99875
  spline S40 degree 3 poles (-11.4806, 27.7163) (-11.6922, 27.6274) (-11.8368, 27.4775) (-11.8992, 27.3735) (-11.9254, 27.3299) (-11.9405, 27.2909) (-11.9492, 27.2619) (-11.954, 27.2455) (-11.9571, 27.2325) (-11.9745, 27.1552) (-11.9853, 27.1068) (-11.9937, 27.0422) (-12.0516, 26.8824) (-12.0928, 26.7687) (-12.1755, 26.5688) (-12.3606, 26.3624) (-12.5062, 26.2) (-12.6843, 26.0846) (-12.7771, 26.0347) (-12.8623, 25.9889) (-12.9316, 25.9512) (-13.1027, 25.9045) (-13.3171, 25.8459) (-13.6108, 25.8438) (-13.7847, 25.875) (-14.1071, 25.933) (-14.173, 25.9939) (-14.2352, 26.0223) (-14.3734, 26.0856) (-14.3508, 26.0762) (-14.3854, 26.0865) (-14.4991, 26.1203) (-14.744, 26.1267) (-15.0001, 25.9807) knots 0.001251 0.001251 0.001251 0.001251 0.25 0.25 0.25 0.35404 0.35404 0.35404 0.412746 0.412746 0.412746 0.449449 0.449449 0.449449 0.475576 0.475576 0.475576 0.496118 0.496118 0.496118 0.514995 0.514995 0.514995 0.538647 0.538647 0.538647 0.582499 0.582499 0.582499 0.679826 0.679826 0.679826 0.99875 0.99875 0.99875 0.99875
  spline S41 degree 3 poles (-15.0001, 25.9807) (-15.1983, 25.8649) (-15.322, 25.6975) (-15.3704, 25.5861) (-15.3906, 25.5395) (-15.4006, 25.4989) (-15.4053, 25.469) (-15.408, 25.4521) (-15.4093, 25.4388) (-15.4165, 25.3599) (-15.421, 25.3105) (-15.4208, 25.2453) (-15.4573, 25.0794) (-15.4834, 24.9613) (-15.5393, 24.7523) (-15.6959, 24.5234) (-15.819, 24.3435) (-15.9805, 24.2058) (-16.066, 24.1443) (-16.1444, 24.0877) (-16.2082, 24.0413) (-16.3718, 23.9726) (-16.5767, 23.8866) (-16.8677, 23.8461) (-17.0441, 23.8544) (-17.3713, 23.8698) (-17.4446, 23.9215) (-17.51, 23.9416) (-17.6553, 23.9863) (-17.6316, 23.9799) (-17.6673, 23.9856) (-17.7844, 24.0044) (-18.028, 23.9787) (-18.2629, 23.8005) knots 0.001251 0.001251 0.001251 0.001251 0.25 0.25 0.25 0.35404 0.35404 0.35404 0.412746 0.412746 0.412746 0.449449 0.449449 0.449449 0.475576 0.475576 0.475576 0.496118 0.496118 0.496118 0.514995 0.514995 0.514995 0.538647 0.538647 0.538647 0.582499 0.582499 0.582499 0.679826 0.679826 0.679826 0.99875 0.99875 0.99875 0.99875
  spline S42 degree 3 poles (-18.2629, 23.8005) (-18.4443, 23.6598) (-18.5451, 23.4777) (-18.5786, 23.361) (-18.5925, 23.3122) (-18.5971, 23.2705) (-18.5979, 23.2403) (-18.5984, 23.2232) (-18.5979, 23.2099) (-18.5947, 23.1307) (-18.5927, 23.0811) (-18.5841, 23.0165) (-18.5986, 22.8472) (-18.609, 22.7267) (-18.6372, 22.5123) (-18.7625, 22.2649) (-18.8611, 22.0704) (-19.0033, 21.9129) (-19.08, 21.8407) (-19.1504, 21.7743) (-19.2076, 21.72) (-19.3608, 21.6306) (-19.5527, 21.5185) (-19.8359, 21.4404) (-20.012, 21.4256) (-20.3383, 21.3981) (-20.4177, 21.4399) (-20.4852, 21.4513) (-20.6351, 21.4766) (-20.6108, 21.4734) (-20.647, 21.4744) (-20.7655, 21.4777) (-21.0037, 21.4205) (-21.2133, 21.2131) knots 0.001251 0.001251 0.001251 0.001251 0.25 0.25 0.25 0.35404 0.35404 0.35404 0.412746 0.412746 0.412746 0.449449 0.449449 0.449449 0.475576 0.475576 0.475576 0.496118 0.496118 0.496118 0.514995 0.514995 0.514995 0.538647 0.538647 0.538647 0.582499 0.582499 0.582499 0.679826 0.679826 0.679826 0.99875 0.99875 0.99875 0.99875
  spline S43 degree 3 poles (-21.2133, 21.2131) (-21.3747, 21.05) (-21.4509, 20.8562) (-21.4688, 20.7361) (-21.4763, 20.6859) (-21.4754, 20.6441) (-21.4722, 20.6139) (-21.4705, 20.5969) (-21.4683, 20.5838) (-21.4548, 20.5057) (-21.4463, 20.4568) (-21.4293, 20.3939) (-21.4217, 20.2242) (-21.4162, 20.1033) (-21.4162, 19.887) (-21.5082, 19.6254) (-21.5805, 19.4198) (-21.701, 19.245) (-21.7675, 19.1634) (-21.8287, 19.0884) (-21.8783, 19.0271) (-22.0185, 18.9184) (-22.1942, 18.7823) (-22.4648, 18.6679) (-22.6374, 18.6302) (-22.9574, 18.5604) (-23.0415, 18.5914) (-23.1099, 18.5939) (-23.2618, 18.5994) (-23.2373, 18.5994) (-23.2733, 18.5957) (-23.3912, 18.5835) (-23.6199, 18.4957) (-23.8007, 18.2627) knots 0.001251 0.001251 0.001251 0.001251 0.25 0.25 0.25 0.35404 0.35404 0.35404 0.412746 0.412746 0.412746 0.449449 0.449449 0.449449 0.475576 0.475576 0.475576 0.496118 0.496118 0.496118 0.514995 0.514995 0.514995 0.538647 0.538647 0.538647 0.582499 0.582499 0.582499 0.679826 0.679826 0.679826 0.99875 0.99875 0.99875 0.99875
  spline S44 degree 3 poles (-23.8007, 18.2627) (-23.9394, 18.0799) (-23.9897, 17.8779) (-23.9918, 17.7565) (-23.9926, 17.7057) (-23.9862, 17.6643) (-23.9792, 17.6349) (-23.9752, 17.6183) (-23.9714, 17.6055) (-23.9478, 17.5298) (-23.933, 17.4825) (-23.908, 17.4224) (-23.8782, 17.2551) (-23.857, 17.136) (-23.8287, 16.9215) (-23.8858, 16.6502) (-23.9307, 16.4368) (-24.0273, 16.2478) (-24.0826, 16.1582) (-24.1335, 16.0759) (-24.1747, 16.0086) (-24.2995, 15.8826) (-24.4559, 15.7247) (-24.7092, 15.576) (-24.8754, 15.5161) (-25.1836, 15.4051) (-25.2711, 15.4249) (-25.3392, 15.4184) (-25.4905, 15.404) (-25.4662, 15.4072) (-25.5014, 15.3988) (-25.6167, 15.3713) (-25.832, 15.2544) (-25.9808, 14.9999) knots 0.001251 0.001251 0.001251 0.001251 0.25 0.25 0.25 0.35404 0.35404 0.35404 0.412746 0.412746 0.412746 0.449449 0.449449 0.449449 0.475576 0.475576 0.475576 0.496118 0.496118 0.496118 0.514995 0.514995 0.514995 0.538647 0.538647 0.538647 0.582499 0.582499 0.582499 0.679826 0.679826 0.679826 0.99875 0.99875 0.99875 0.99875
  spline S45 degree 3 poles (-25.9808, 14.9999) (-26.0945, 14.8005) (-26.118, 14.5936) (-26.1042, 14.473) (-26.0984, 14.4226) (-26.0867, 14.3824) (-26.0759, 14.3541) (-26.0698, 14.3382) (-26.0643, 14.326) (-26.031, 14.2541) (-26.0102, 14.2091) (-25.9775, 14.1527) (-25.9262, 13.9907) (-25.8896, 13.8754) (-25.8336, 13.6665) (-25.8547, 13.39) (-25.8714, 13.1726) (-25.9425, 12.9726) (-25.9857, 12.8766) (-26.0253, 12.7883) (-26.0574, 12.7162) (-26.1647, 12.575) (-26.2992, 12.398) (-26.5309, 12.2175) (-26.6879, 12.1364) (-26.9789, 11.9862) (-27.0682, 11.9944) (-27.135, 11.9791) (-27.2831, 11.9451) (-27.2594, 11.9514) (-27.2932, 11.9385) (-27.4039, 11.8962) (-27.6021, 11.7522) (-27.7164, 11.4804) knots 0.001251 0.001251 0.001251 0.001251 0.25 0.25 0.25 0.35404 0.35404 0.35404 0.412746 0.412746 0.412746 0.449449 0.449449 0.449449 0.475576 0.475576 0.475576 0.496118 0.496118 0.496118 0.514995 0.514995 0.514995 0.538647 0.538647 0.538647 0.582499 0.582499 0.582499 0.679826 0.679826 0.679826 0.99875 0.99875 0.99875 0.99875
  spline S46 degree 3 poles (-27.7164, 11.4804) (-27.8031, 11.2679) (-27.7994, 11.0597) (-27.77, 10.9419) (-27.7577, 10.8927) (-27.7408, 10.8543) (-27.7264, 10.8277) (-27.7182, 10.8127) (-27.7112, 10.8014) (-27.6688, 10.7344) (-27.6423, 10.6925) (-27.6025, 10.6409) (-27.5305, 10.487) (-27.4792, 10.3774) (-27.3964, 10.1776) (-27.3813, 9.9007) (-27.3694, 9.683) (-27.4138, 9.4754) (-27.4441, 9.3746) (-27.4719, 9.2819) (-27.4943, 9.2063) (-27.5822, 9.0522) (-27.6924, 8.8592) (-27.8986, 8.65) (-28.0437, 8.5492) (-28.3126, 8.3622) (-28.4022, 8.3586) (-28.4664, 8.3347) (-28.6088, 8.2817) (-28.5861, 8.2911) (-28.618, 8.2739) (-28.7223, 8.2175) (-28.8999, 8.0488) (-28.9778, 7.7644) knots 0.001251 0.001251 0.001251 0.001251 0.25 0.25 0.25 0.35404 0.35404 0.35404 0.412746 0.412746 0.412746 0.449449 0.449449 0.449449 0.475576 0.475576 0.475576 0.496118 0.496118 0.496118 0.514995 0.514995 0.514995 0.538647 0.538647 0.538647 0.582499 0.582499 0.582499 0.679826 0.679826 0.679826 0.99875 0.99875 0.99875 0.99875
  spline S47 degree 3 poles (-28.9778, 7.7644) (-29.036, 7.5424) (-29.0052, 7.3365) (-28.9606, 7.2236) (-28.942, 7.1764) (-28.9203, 7.1406) (-28.9025, 7.1161) (-28.8924, 7.1022) (-28.884, 7.0919) (-28.8332, 7.031) (-28.8015, 6.993) (-28.7553, 6.947) (-28.6638, 6.8038) (-28.5987, 6.7019) (-28.4905, 6.5146) (-28.4393, 6.242) (-28.3991, 6.0278) (-28.4161, 5.8162) (-28.4329, 5.7122) (-28.4484, 5.6167) (-28.4607, 5.5388) (-28.5278, 5.3746) (-28.6119, 5.1689) (-28.789, 4.9345) (-28.9196, 4.8156) (-29.1619, 4.5951) (-29.2503, 4.5799) (-29.3108, 4.5478) (-29.445, 4.4767) (-29.4238, 4.4889) (-29.4531, 4.4677) (-29.5491, 4.3982) (-29.7033, 4.2078) (-29.7434, 3.9157) knots 0.001251 0.001251 0.001251 0.001251 0.25 0.25 0.25 0.35404 0.35404 0.35404 0.412746 0.412746 0.412746 0.449449 0.449449 0.449449 0.475576 0.475576 0.475576 0.496118 0.496118 0.496118 0.514995 0.514995 0.514995 0.538647 0.538647 0.538647 0.582499 0.582499 0.582499 0.679826 0.679826 0.679826 0.99875 0.99875 0.99875 0.99875
  dimension "d64" = 16
  dimension "d65" = 10
  dimension "d66" = 15
  dimension "d68" = 360
  constraint coincident A0.centre origin
  constraint horizontal A0.centre A1.centre
  measures "d64" diameter of A0
  measures "d65" diameter of A1
  measures "d66" distance of A0.centre A1.centre
extrude "Extrude2" cut sketch "Sketch2" against normal blind 6 contours A0 | A1 | A2 | A3 | A4 | A5